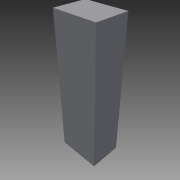
# Autodesk Inventor part: test string
Saved by Autodesk Inventor 2013 (Build 170138000, 138)
## iProperties
Created: 2014-06-22
Part Number: test string
Material: Generic
Document SubType Name: Modeling
Designer: employee
Density: 1 g/cm^3
Author: employee
Autodesk Inventor part; units mm, degrees
ref_plane "YZ Plane" through (0, 0, 0) normal (1, 0, 0) x (0, 1, 0)
ref_plane "XZ Plane" through (0, 0, 0) normal (0, 1, 0) x (-1, 0, 0)
ref_plane "XY Plane" through (0, 0, 0) normal (0, 0, 1) x (1, 0, 0)
sketch "Sketch1" plane through (0, 0, 0) normal (0, 0, 1) x (1, 0, 0)
  line L0 (-47.9982, 21.4874) -> (268.0018, 21.4874) projected
  line L1 (-26.4982, 131.0411) -> (246.5018, 131.0411) projected
  line L2 (110.0018, 131.0411) -> (76.2689, 131.0411)
  line L3 (76.2689, 131.0411) -> (76.2689, 21.4874)
  line L4 (76.2689, 21.4874) -> (110.0018, 21.4874)
  line L5 (110.0018, 21.4874) -> (110.0018, 131.0411)
  point P0 (0, 0)
  constraints: 8 end point, 2 parallel, 1 horizontal, 1 midpoint, 1 perpendicular, 1 point on line
extrude "Extrusion1" add sketch "Sketch1" along normal blind 25.4
body "Solid1"
